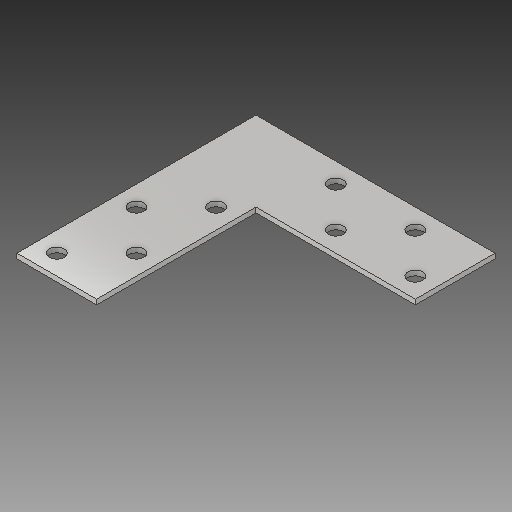
# Autodesk Inventor part: elvRivetPlate
Saved by Autodesk Inventor 2019 (Build 230136000, 136)
## iProperties
Created: 2019-01-16
Part Number: elvRivetPlate
Material: Generic
Document SubType Name: Modeling
Designer: james
Density: 1 g/cm^3
Appearance: Aluminum - Polished
Mass: 4.89472 g
Surface Area: 68.4046 cm^2
Volume: 4.89472 cm^3
Author: james
Autodesk Inventor part; units mm, degrees
ref_plane "YZ Plane" through (0, 0, 0) normal (1, 0, 0) x (0, 1, 0)
ref_plane "XZ Plane" through (0, 0, 0) normal (0, 1, 0) x (-1, 0, 0)
ref_plane "XY Plane" through (0, 0, 0) normal (0, 0, 1) x (1, 0, 0)
sketch "Sketch1" plane through (0, 0, 0) normal (0, 1, 0) x (-1, 0, 0)
  line L0 (46.3062, 23.9021) -> (20.9062, 23.9021)
  line L1 (20.9062, 23.9021) -> (20.9062, -26.8979)
  line L2 (15.3051, -52.2979) -> (46.3062, -52.2979)
  line L3 (46.3062, -52.2979) -> (46.3062, 23.9021)
  line L4 (46.3062, -52.2979) -> (-29.8938, -52.2979)
  line L5 (-29.8938, -52.2979) -> (-29.8938, -26.8979)
  line L6 (-29.8938, -26.8979) -> (20.9062, -26.8979)
  line L7 (46.3062, -26.8979) -> (46.3062, -52.2979)
  point P0 (0, 0)
  dimension "d0" = 25.4
  dimension "d1" = 25.4
  dimension "d2" = 76.2
  dimension "d3" = 76.2
  constraints: 16 end point, 4 parallel, 2 horizontal, 2 perpendicular
  measures "d0" distance between parallel lines of L4 L6
  measures "d1" distance between parallel lines of L1 L3
  measures "d2" distance between parallel lines of L2 L0
  measures "d3" distance between parallel lines of L5 L3
extrude "Extrusion1" add sketch "Sketch1" along normal blind 1.5875
sketch "Sketch2" plane through (0, 1.5875, 0) normal (0, 1, 0) x (1, 0, 0)
  line L0 (-46.3062, -23.9021) -> (-20.9062, -23.9021) projected
  line L1 (-46.3062, 52.2979) -> (-46.3062, -23.9021) projected
  line L2 (-20.9062, -23.9021) -> (-20.9062, 26.8979) projected
  point P0 (0, 0)
  point P1 (-39.9562, -17.5521)
  point P2 (-27.2562, -4.8521)
  point P3 (-39.9562, 7.8479)
  point P4 (-27.2562, 20.5479)
  dimension "d6" = 6.35
  dimension "d7" = 6.35
  dimension "d8" = 6.35
  dimension "d9" = 12.7
  dimension "d10" = 12.7
  dimension "d11" = 6.35
  dimension "d12" = 12.7
  dimension "d13" = 6.35
  measures "d6" distance from line of L0 point (-39.956, -17.552)
  measures "d7" distance from line of L1 point (-39.956, -17.552)
  measures "d8" distance from line of L2 point (-27.256, -4.852)
  measures "d9" horizontal distance of point (-39.956, -17.552) point (-27.256, -4.852)
  measures "d10" horizontal distance of point (-27.256, -4.852) point (-39.956, 7.848)
  measures "d11" distance from line of L1 point (-39.956, 7.848)
  measures "d12" horizontal distance of point (-39.956, 7.848) point (-27.256, 20.548)
  measures "d13" distance from line of L2 point (-27.256, 20.548)
hole "Hole1" at (-39.9562, 1.5875, 17.5521) at (-27.2562, 1.5875, 4.8521) at (-39.9562, 1.5875, -7.8479) at (-27.2562, 1.5875, -20.5479) direction (0, -1, 0) diameter 4.7625 depth 25.4 tip angle 118
sketch "Sketch3" plane through (0, 1.5875, 0) normal (0, 1, 0) x (1, 0, 0)
  line L0 (29.8938, 26.8979) -> (29.8938, 52.2979) projected
  line L1 (-20.9062, 26.8979) -> (29.8938, 26.8979) projected
  line L2 (29.8938, 52.2979) -> (-46.3062, 52.2979) projected
  point P0 (0, 0)
  point P1 (-14.5562, 45.9479)
  point P2 (-1.8562, 33.2479)
  point P3 (23.5438, 33.2479)
  point P4 (10.8438, 45.9479)
  dimension "d21" = 6.35
  dimension "d22" = 6.35
  dimension "d23" = 12.7
  dimension "d24" = 6.35
  dimension "d25" = 12.7
  dimension "d26" = 6.35
  dimension "d27" = 12.7
  dimension "d28" = 6.35
  measures "d21" distance from line of L0 point (23.544, 33.248)
  measures "d22" distance from line of L1 point (23.544, 33.248)
  measures "d23" horizontal distance of point (23.544, 33.248) point (10.844, 45.948)
  measures "d24" distance from line of L2 point (10.844, 45.948)
  measures "d25" horizontal distance of point (-1.856, 33.248) point (10.844, 45.948)
  measures "d26" distance from line of L1 point (-1.856, 33.248)
  measures "d27" horizontal distance of point (-14.556, 45.948) point (-1.856, 33.248)
  measures "d28" distance from line of L2 point (-14.556, 45.948)
hole "Hole2" at (-14.5562, 1.5875, -45.9479) at (-1.8562, 1.5875, -33.2479) at (23.5438, 1.5875, -33.2479) at (10.8438, 1.5875, -45.9479) direction (0, -1, 0) diameter 4.7625 depth 25.4 tip angle 118
equation "\"d0\" = ElvBeamWidth"
equation "\"d1\" = ElvBeamWidth"
equation "\"d2\" = ElvRivetPlateLength"
equation "\"d3\" = ElvRivetPlateLength"
equation "\"d4\" = ElvWallWidth"
equation "\"ElvCrossBeamLength\" = 304.8"
equation "\"ElvFixedBeamLength\" = 990.6"
equation "\"ElvMiddleBeamLength\" = 990.6"
equation "\"ElvFrontBeamLength\" = 990.6"
equation "\"ElvEndEffectLength\" = 431.8"
equation "\"ElvBeamWidth\" = 25.4"
equation "\"ElvWallWidth\" = 1.5875"
equation "\"ElvDelWidth\" = 18.542"
equation "\"ElvDelHeight\" = 101.6"
equation "\"ElvDelFrontTabLength\" = 6.35"
equation "\"ElvDelDepth\" = 6.35"
equation "\"ElvTopBeamLength\" = 457.2"
equation "\"ElvHoleFromFront\" = 25.4"
equation "\"ElvHoleFromMid\" = 38.1"
equation "\"ElvHoleFromFixed\" = 50.8"
equation "\"ElvHoleFromBottom\" = 38.1"
equation "\"ElvRivetPlateLength\" = 76.2"
equation "\"ElvDelMiddleTabLength\" = 6.35"
body "Solid1"
